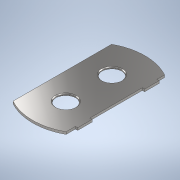
# Autodesk Inventor part: VR_Cam_Kismi
Saved by Autodesk Inventor 2022 (Build 260153070, 153G)
## iProperties
Created: 2021-10-26
Part Number: VR_Cam_Kismi
Material: Stainless Steel, Austenitic
Document SubType Name: Modeling
Designer: doguh
Density: 8 g/cm^3
Appearance: Semi-Polished
Author: doguh
## iProperties of the stored document VR_Cam_Kismi_3DPrint.ipt
Created: 2021-10-26
Part Number: VR_Cam_Kismi_3DPrint
Material: Generic
Document SubType Name: Modeling
Designer: doguh
Density: 1 g/cm^3
Appearance: Default
Author: doguh
Autodesk Inventor part; units mm, degrees
ref_plane "YZ Plane" through (0, 0, 0) normal (1, 0, 0) x (0, 1, 0)
ref_plane "XZ Plane" through (0, 0, 0) normal (0, 1, 0) x (-1, 0, 0)
ref_plane "XY Plane" through (0, 0, 0) normal (0, 0, 1) x (1, 0, 0)
sketch "Sketch1" plane through (0, 0, 0) normal (0, 1, 0) x (-1, 0, 0)
  line L0 (34.4615, 64) -> (34.4615, -64)
  line L1 (-34.4615, -64) -> (-34.4615, 64)
  line L2 (-34.4615, 64) -> (34.4615, -64) construction
  line L3 (34.4615, 64) -> (-34.4615, -64) construction
  arc A0 (-34.4615, -64) -> (34.4615, -64) centre (0, -1.4222) ccw
  arc A1 (34.4615, 64) -> (-34.4615, 64) centre (0, 1.4222) ccw
  point P0 (0, 0)
  dimension "d1" = 128
  constraints: 8 end point, 4 point on circle, 2 centre point, 2 midpoint, 1 parallel
  measures "d1" distance of L0.start L0.end
extrude "taban" add sketch "Sketch1" along normal blind 3
sketch "Sketch2" plane through (0, 3, 0) normal (0, 1, 0) x (1, 0, 0)
  circle A0 centre (0, 30) radius 12.5
  circle A1 centre (0, -30) radius 12.5
  constraints: 2 centre point
extrude "cam" cut sketch "Sketch2" against normal blind 3
sketch "Sketch3" plane through (34.4615, 0, 64) normal (1, 0, 0) x (0, 0, -1)
  line L0 (12, 3) -> (31, 3)
  line L1 (31, 3) -> (31, 0)
  line L2 (31, 0) -> (12, 0)
  line L3 (12, 0) -> (12, 3)
  line L4 (118, 3) -> (99, 3)
  line L5 (99, 3) -> (99, 0)
  line L6 (99, 0) -> (118, 0)
  line L7 (118, 0) -> (118, 3)
  constraints: 16 end point, 4 parallel, 2 horizontal, 2 perpendicular
extrude "sikigecme" add sketch "Sketch3" along normal blind 3
chamfer "Chamfer1" distance 1 angle 45 4 edges at (-12.5, 0, -30) (-12.5, 0, 30) (-12.5, 3, 30) (-12.5, 3, -30)
body "Solid1"
